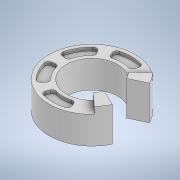
# Autodesk Inventor part: pawn
Saved by Autodesk Inventor 2021.1 (Build 251245010, 245A)
## iProperties
Created: 2021-09-08
Part Number: pawn
Material: Типовые
Document SubType Name: Modeling
Designer: User
Density: 1 g/cm^3
Appearance: По умолчанию
Author: User
Autodesk Inventor part; units mm, degrees
ref_plane "YZ Plane" through (0, 0, 0) normal (1, 0, 0) x (0, 1, 0)
ref_plane "XZ Plane" through (0, 0, 0) normal (0, 1, 0) x (-1, 0, 0)
ref_plane "XY Plane" through (0, 0, 0) normal (0, 0, 1) x (1, 0, 0)
sketch "Эскиз1" plane through (0, 0, 0) normal (0, 1, 0) x (-1, 0, 0)
  arc A0 (-11.2808, -5.3845) -> (-11.2808, 5.3845) centre (0, 0) ccw
  arc A1 (-6.7685, -3.2307) -> (-6.7685, 3.2307) centre (0, 0) ccw
  line L0 (-6.7685, -3.2307) -> (-11.2808, -5.3845)
  line L1 (-6.7685, 3.2307) -> (-11.2808, 5.3845)
  dimension "d0" = 25
  dimension "d1" = 15
  constraints: 4 end point, 4 point on circle, 2 centre point, 2 coincident
  measures "d0" diameter of A0
  measures "d1" diameter of A1
extrude "Выдавливание1" add sketch "Эскиз1" along normal blind 8
sketch "Эскиз2" plane through (0, 8, 0) normal (0, 1, 0) x (1, 0, 0)
  line L0 (5.4983, 5.1008) -> (9.1638, 8.5014)
  arc A0 (11.2808, 5.3845) -> (11.2808, -5.3845) centre (0, 0) ccw projected
  arc A1 (11.2808, 5.3845) -> (11.2808, -5.3845) centre (0, 0) ccw projected
  line L1 (11.2808, -5.3845) -> (6.7685, -3.2307) projected
  arc A2 (6.7685, 3.2307) -> (6.7685, -3.2307) centre (0, 0) ccw projected
  line L2 (6.7685, 3.2307) -> (11.2808, 5.3845) projected
  arc A3 (6.7685, 3.2307) -> (6.7685, -3.2307) centre (0, 0) ccw projected
  line L3 (5.4983, -5.1008) -> (9.1638, -8.5014)
  point P0 (11.2808, -5.3845)
  constraints: 4 end point, 1 point on circle
extrude "Выдавливание2" add sketch "Эскиз2" along normal blind 2 contours L0 A0 L2 A2 | A2 L1 A0 L3
sketch "Эскиз3" plane through (0, 8, 0) normal (0, 1, 0) x (1, 0, 0)
  arc A0 (2.2493, 8.197) -> (-2.2493, 8.197) centre (0, 0) ccw
  arc A1 (3.1548, 11.0588) -> (-3.1548, 11.0588) centre (0, 0) ccw
  line L0 (3.4451, 8.7967) -> (3.8116, 9.7325)
  arc A2 (9.1638, 8.5014) -> (9.1638, -8.5014) centre (0, 0) ccw projected
  arc A3 (5.4983, 5.1008) -> (5.4983, -5.1008) centre (0, 0) ccw projected
  line L1 (-3.4451, 8.7967) -> (-3.8116, 9.7325)
  arc A4 (3.8116, 9.7325) -> (3.1548, 11.0588) centre (2.8804, 10.0972) ccw
  arc A5 (2.2493, 8.197) -> (3.4451, 8.7967) centre (2.5139, 9.1613) ccw
  arc A6 (-3.1548, 11.0588) -> (-3.8116, 9.7325) centre (-2.8804, 10.0972) ccw
  arc A7 (-3.4451, 8.7967) -> (-2.2493, 8.197) centre (-2.5139, 9.1613) ccw
  arc A8 (-5.9741, 6.0464) -> (-5.8956, 7.3819) centre (-6.677, 6.7578) ccw
  line L2 (-5.8956, 7.3819) -> (-6.5228, 8.1672)
  arc A9 (-5.9741, 6.0464) -> (-8.2235, 2.1505) centre (0, 0) ccw
  arc A10 (-9.3407, 1.4148) -> (-8.2235, 2.1505) centre (-9.1909, 2.4035) ccw
  arc A11 (-6.5228, 8.1672) -> (-7.9998, 8.2615) centre (-7.3042, 7.5431) ccw
  line L3 (-9.3407, 1.4148) -> (-10.3344, 1.5653)
  arc A12 (-11.1546, 2.7973) -> (-10.3344, 1.5653) centre (-10.1846, 2.5541) ccw
  arc A13 (-7.9998, 8.2615) -> (-11.1546, 2.7973) centre (0, 0) ccw
  arc A14 (-8.2235, -2.1505) -> (-9.3407, -1.4148) centre (-9.1909, -2.4035) ccw
  line L4 (-9.3407, -1.4148) -> (-10.3344, -1.5653)
  arc A15 (-8.2235, -2.1505) -> (-5.9741, -6.0464) centre (0, 0) ccw
  arc A16 (-5.8956, -7.3819) -> (-5.9741, -6.0464) centre (-6.677, -6.7578) ccw
  arc A17 (-10.3344, -1.5653) -> (-11.1546, -2.7973) centre (-10.1846, -2.5541) ccw
  line L5 (-5.8956, -7.3819) -> (-6.5228, -8.1672)
  arc A18 (-7.9998, -8.2615) -> (-6.5228, -8.1672) centre (-7.3042, -7.5431) ccw
  arc A19 (-11.1546, -2.7973) -> (-7.9998, -8.2615) centre (0, 0) ccw
  arc A20 (-2.2493, -8.197) -> (-3.4451, -8.7967) centre (-2.5139, -9.1613) ccw
  line L6 (-3.4451, -8.7967) -> (-3.8116, -9.7325)
  arc A21 (-2.2493, -8.197) -> (2.2493, -8.197) centre (0, 0) ccw
  arc A22 (3.4451, -8.7967) -> (2.2493, -8.197) centre (2.5139, -9.1613) ccw
  arc A23 (-3.8116, -9.7325) -> (-3.1548, -11.0588) centre (-2.8804, -10.0972) ccw
  line L7 (3.4451, -8.7967) -> (3.8116, -9.7325)
  arc A24 (3.1548, -11.0588) -> (3.8116, -9.7325) centre (2.8804, -10.0972) ccw
  arc A25 (-3.1548, -11.0588) -> (3.1548, -11.0588) centre (0, 0) ccw
  point P0 (4.1936, 10.7081)
  point P1 (3.0996, 7.9147)
  point P2 (-4.1936, 10.7081)
  point P3 (-3.0996, 7.9147)
  point P4 (-5.3045, 6.6417)
  point P5 (-8.4041, 1.273)
  point P6 (-7.1767, 8.9859)
  point P7 (-11.3703, 1.7222)
  point P8 (-8.4041, -1.273)
  point P9 (-5.3045, -6.6417)
  point P10 (-11.3703, -1.7222)
  point P11 (-7.1767, -8.9859)
  point P12 (-3.0996, -7.9147)
  point P13 (3.0996, -7.9147)
  point P14 (-4.1936, -10.7081)
  point P15 (4.1936, -10.7081)
  dimension "d8" = 3
  dimension "d9" = 1
  dimension "d12" = 180
  constraints: 64 point on circle, 24 centre point, 16 end point, 16 point on line, 8 tangent, 5 coincident, 3 equal radius, 79 other
  measures "d8" radial gap between concentric circles of A0 A1
  measures "d9" radius of A4
extrude "Выдавливание3" cut sketch "Эскиз3" against normal blind 1
